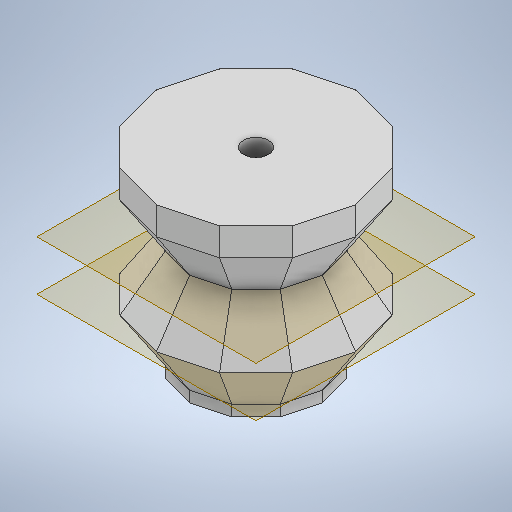
# Autodesk Inventor part: diameter36mm
Saved by Autodesk Inventor 2025.1 (Build 291241000, 241)
## iProperties
Created: 2024-08-08
Part Number: diameter36mm
Material: 일반
Document SubType Name: Modeling
Designer: 82103
Density: 1 g/cm^3
Appearance: 기본값
Author: 82103
Autodesk Inventor part; units mm, degrees
ref_plane "YZ Plane" through (0, 0, 0) normal (1, 0, 0) x (0, 1, 0)
ref_plane "XY Plane" through (0, 0, 0) normal (0, 0, 1) x (1, 0, 0)
sketch "스케치1" plane through (0, 0, 0) normal (0, 1, 0) x (-1, 0, 0)
  line L0 (15.5885, -9) -> (9, -15.5885)
  line L1 (9, -15.5885) -> (0, -18)
  line L2 (0, -18) -> (-9, -15.5885)
  line L3 (-9, -15.5885) -> (-15.5885, -9)
  line L4 (-15.5885, -9) -> (-18, 0)
  line L5 (-18, 0) -> (-15.5885, 9)
  line L6 (-15.5885, 9) -> (-9, 15.5885)
  line L7 (-9, 15.5885) -> (0, 18)
  line L8 (0, 18) -> (9, 15.5885)
  line L9 (9, 15.5885) -> (15.5885, 9)
  line L10 (15.5885, 9) -> (18, 0)
  line L11 (18, 0) -> (15.5885, -9)
  point P0 (0, 0)
  point P1 (0, 0)
  dimension "d0" = 36
  constraints: 24 end point, 1 coincident, 1 vertical alignment, 25 other
  measures "d0" distance of L4.end L10.end
ref_plane "작업 평면1" through (0, 9, 0) normal (0, 1, 0) x (-1, 0, 0)
sketch "스케치2" plane through (0, 9, 0) normal (0, 1, 0) x (-1, 0, 0)
  line L0 (10.3923, -6) -> (6, -10.3923)
  line L1 (6, -10.3923) -> (0, -12)
  line L2 (0, -12) -> (-6, -10.3923)
  line L3 (-6, -10.3923) -> (-10.3923, -6)
  line L4 (-10.3923, -6) -> (-12, 0)
  line L5 (-12, 0) -> (-10.3923, 6)
  line L6 (-10.3923, 6) -> (-6, 10.3923)
  line L7 (-6, 10.3923) -> (0, 12)
  line L8 (0, 12) -> (6, 10.3923)
  line L9 (6, 10.3923) -> (10.3923, 6)
  line L10 (10.3923, 6) -> (12, 0)
  line L11 (12, 0) -> (10.3923, -6)
  point P0 (0, 0)
  point P1 (0, 0)
  dimension "d2" = 24
  constraints: 24 end point, 1 coincident, 1 vertical alignment, 25 other
  measures "d2" distance of L4.end L10.end
loft "로프트1" add profiles "스케치2", "스케치1"
mirror "미러1" about plane through (0, 9, 0) normal (0, 1, 0) of "로프트1"
mirror "미러2" about plane through (0, 0, 0) normal (0, 1, 0) of "로프트1"
sketch "스케치3" plane through (-6, -9, -10.3923) normal (0, -1, 0) x (0.7071068, 0, 0.7071068)
  line L0 (8.4853, -8.4853) -> (14.6969, -8.4853) projected
  line L1 (3.1058, -5.3795) -> (8.4853, -8.4853) projected
  line L2 (0, 0) -> (3.1058, -5.3795) projected
  line L3 (0, 6.2117) -> (0, 0) projected
  line L4 (3.1058, 11.5911) -> (0, 6.2117) projected
  line L5 (8.4853, 14.6969) -> (3.1058, 11.5911) projected
  line L6 (14.6969, 14.6969) -> (8.4853, 14.6969) projected
  line L7 (20.0764, 11.5911) -> (14.6969, 14.6969) projected
  line L8 (23.1822, 6.2117) -> (20.0764, 11.5911) projected
  line L9 (23.1822, 0) -> (23.1822, 6.2117) projected
  line L10 (20.0764, -5.3795) -> (23.1822, 0) projected
  line L11 (0, 6.2117) -> (0, 0) projected
  line L12 (0, 0) -> (3.1058, -5.3795) projected
  line L13 (3.1058, -5.3795) -> (8.4853, -8.4853) projected
  line L14 (8.4853, -8.4853) -> (14.6969, -8.4853) projected
  line L15 (14.6969, -8.4853) -> (20.0764, -5.3795) projected
  line L16 (20.0764, -5.3795) -> (23.1822, 0) projected
  line L17 (23.1822, 0) -> (23.1822, 6.2117) projected
  line L18 (23.1822, 6.2117) -> (20.0764, 11.5911) projected
  line L19 (20.0764, 11.5911) -> (14.6969, 14.6969) projected
  line L20 (14.6969, 14.6969) -> (8.4853, 14.6969) projected
  line L21 (8.4853, 14.6969) -> (3.1058, 11.5911) projected
  line L22 (3.1058, 11.5911) -> (0, 6.2117) projected
  point P0 (11.5911, 3.1058)
  point P1 (14.6969, -8.4853)
shell "쉘1" thickness 0.5 removed faces 0 ; own thickness 2 on faces at (-15.8612, -1.5, 4.25) (-11.6112, -1.5, 11.6112) (-15.8612, -1.5, -4.25) (-11.6112, -1.5, -11.6112) (-4.25, -1.5, 15.8612) (4.25, -1.5, 15.8612) (11.6112, -1.5, 11.6112) (15.8612, -1.5, 4.25) (15.8612, -1.5, -4.25) (11.6112, -1.5, -11.6112) (4.25, -1.5, -15.8612) (-4.25, -1.5, -15.8612) (-15.8612, 16.5, -4.25) (-15.8612, 16.5, 4.25) (-11.6112, 16.5, 11.6112) (-11.6112, 16.5, -11.6112) (-4.25, 16.5, 15.8612) (4.25, 16.5, 15.8612) (11.6112, 16.5, 11.6112) (15.8612, 16.5, 4.25) (15.8612, 16.5, -4.25) (11.6112, 16.5, -11.6112) (4.25, 16.5, -15.8612) (-4.25, 16.5, -15.8612)
extrude "돌출1" add sketch "스케치3" along normal blind 2
sketch "스케치4" plane through (-15.5885, 18, -9) normal (0, 1, 0) x (0.7071068, 0, 0.7071068)
  line L0 (12.7279, 22.0454) -> (22.0454, 22.0454) projected
  line L1 (22.0454, 22.0454) -> (30.1146, 17.3867) projected
  line L2 (30.1146, 17.3867) -> (34.7733, 9.3175) projected
  line L3 (34.7733, 9.3175) -> (34.7733, 0) projected
  line L4 (34.7733, 0) -> (30.1146, -8.0692) projected
  line L5 (30.1146, -8.0692) -> (22.0454, -12.7279) projected
  line L6 (22.0454, -12.7279) -> (12.7279, -12.7279) projected
  line L7 (12.7279, -12.7279) -> (4.6587, -8.0692) projected
  line L8 (4.6587, -8.0692) -> (0, 0) projected
  line L9 (0, 0) -> (0, 9.3175) projected
  line L10 (0, 9.3175) -> (4.6587, 17.3867) projected
  line L11 (4.6587, 17.3867) -> (12.7279, 22.0454) projected
  point P0 (17.3867, 4.6587)
extrude "돌출2" add sketch "스케치4" along normal blind 5
sketch "스케치5" plane through (-15.5885, 23, -9) normal (0, 1, 0) x (0.7071068, 0, -0.7071068)
  circle A0 centre (4.6587, -17.3867) radius 2.25
  dimension "d13" = 4.5
  constraints: 1 centre point, 1 coincident
  measures "d13" diameter of A0
extrude "돌출3" cut sketch "스케치5" against normal blind 5.5
